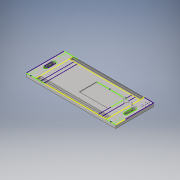
# Autodesk Inventor part: Button Fixture Base
Saved by Autodesk Inventor 2016 (Build 200138000, 138)
## iProperties
Created: 2016-07-07
Part Number: Button Fixture Base
Material: Generic
Document SubType Name: Modeling
Designer: Sam Clay
Density: 1 g/cm^3
Appearance: Default
Author: Sam Clay
Autodesk Inventor part; units mm, degrees
ref_plane "YZ Plane" through (0, 0, 0) normal (1, 0, 0) x (0, 1, 0)
ref_plane "XZ Plane" through (0, 0, 0) normal (0, 1, 0) x (-1, 0, 0)
ref_plane "XY Plane" through (0, 0, 0) normal (0, 0, 1) x (1, 0, 0)
sketch "Sketch1" plane through (0, 0, 0) normal (0, 1, 0) x (-1, 0, 0)
  line L0 (0, 0) -> (381, 0)
  line L1 (381, 0) -> (381, 203.2)
  line L2 (381, 203.2) -> (0, 203.2)
  line L3 (0, 203.2) -> (0, 0)
  line L4 (381, 0) -> (431.8, 0)
  line L5 (431.8, 0) -> (431.8, 203.2)
  line L6 (431.8, 203.2) -> (381, 203.2)
  line L7 (381, 203.2) -> (381, 0)
  line L8 (0, 0) -> (-50.8, 0)
  line L9 (-50.8, 0) -> (-50.8, 203.2)
  line L10 (-50.8, 203.2) -> (0, 203.2)
  line L11 (0, 203.2) -> (0, 0)
  dimension "d0" = 381
  dimension "d1" = 203.2
  dimension "d2" = 50.8
  dimension "d3" = 50.8
  constraints: 24 end point, 6 parallel, 3 horizontal, 3 perpendicular, 2 point on line
  measures "d0" distance of L2.end L1.end
  measures "d1" distance of L1.end L0.end
  measures "d2" distance of L6.end L5.end
  measures "d3" distance of L9.end L10.end
extrude "Extrusion1" add sketch "Sketch1" along normal blind 19.05 contours L3 L2 L1 L0
extrude "Extrusion2" add sketch "Sketch1" along normal blind 17.78 contours L8 L9 L10 L3 | L1 L6 L5 L4
sketch "Sketch2" plane through (0, 19.05, 0) normal (0, 1, 0) x (1, 0, 0)
  line L0 (-381, 0) -> (-381, -203.2) projected
  line L1 (0, 0) -> (-381, 0)
  line L2 (-381, 0) -> (-381, -3.175)
  line L3 (-381, -3.175) -> (0, -3.175)
  line L4 (0, -3.175) -> (0, 0)
  line L5 (0, -3.175) -> (-381, -3.175)
  line L6 (-381, -3.175) -> (-381, -22.987)
  line L7 (-381, -22.987) -> (0, -22.987)
  line L8 (0, -22.987) -> (0, -3.175)
  line L9 (0, -22.987) -> (-381, -22.987)
  line L10 (-381, -22.987) -> (-381, -54.737)
  line L11 (-381, -54.737) -> (0, -54.737)
  line L12 (0, -54.737) -> (0, -22.987)
  line L13 (0, -54.737) -> (-381, -54.737)
  line L14 (-381, -54.737) -> (-381, -148.717)
  line L15 (-381, -148.717) -> (0, -148.717)
  line L16 (0, -148.717) -> (0, -54.737)
  line L17 (0, -148.717) -> (-381, -148.717)
  line L18 (-381, -148.717) -> (-381, -180.467)
  line L19 (-381, -180.467) -> (0, -180.467)
  line L20 (0, -180.467) -> (0, -148.717)
  line L21 (0, -180.467) -> (-381, -180.467)
  line L22 (-381, -180.467) -> (-381, -200.279)
  line L23 (-381, -200.279) -> (0, -200.279)
  line L24 (0, -200.279) -> (0, -180.467)
  line L25 (0, -200.279) -> (-381, -200.279)
  line L26 (-381, -200.279) -> (-381, -203.454)
  line L27 (-381, -203.454) -> (0, -203.454)
  line L28 (0, -203.454) -> (0, -200.279)
  line L29 (0, -203.2) -> (0, 0) projected
  line L30 (0, 0) -> (-44.45, 0)
  line L31 (-44.45, 0) -> (-44.45, -148.717)
  line L32 (-44.45, -148.717) -> (0, -148.717)
  line L33 (0, -148.717) -> (0, 0)
  circle A0 centre (-48.1046, -57.912) radius 8.89
  line L34 (-44.45, -54.737) -> (-199.39, -54.737)
  line L35 (-199.39, -54.737) -> (-199.39, -148.717)
  line L36 (-199.39, -148.717) -> (-44.45, -148.717)
  line L37 (-44.45, -148.717) -> (-44.45, -54.737)
  dimension "d8" = 3.175
  dimension "d9" = 19.812
  dimension "d10" = 31.75
  dimension "d11" = 93.98
  dimension "d12" = 31.75
  dimension "d13" = 19.812
  dimension "d14" = 3.175
  dimension "d15" = 44.45
  dimension "d16" = 17.78
  dimension "d21" = 3.175
  dimension "d49" = 154.94
  constraints: 72 end point, 18 parallel, 11 point on line, 9 horizontal, 9 perpendicular, 1 centre point
  measures "d8" distance of L2.end L1.end
  measures "d9" distance of L6.end L5.end
  measures "d10" distance of L10.end L9.end
  measures "d11" distance of L14.end L13.end
  measures "d12" distance of L18.end L17.end
  measures "d13" distance of L22.end L21.end
  measures "d14" distance of L26.end L25.end
  measures "d15" distance of L32.end L31.end
  measures "d16" diameter of A0
  measures "d21" distance from line of L13 A0.centre
  measures "d49" distance of L36.end L35.end
extrude "Extrusion3" cut sketch "Sketch2" against normal blind 11.43 contours L3 L31 L7 L0 | L3 L8 L7 L31 | L19 L24 L23 L0
extrude "Extrusion4" cut sketch "Sketch2" against normal blind 1.651 contours L11 A0 L31 L15 L35 | A0 L11 L31 | L31 L11 A0 | L11 L31 A0 | L11 A0 L31
sketch "Sketch3" plane through (0, 19.05, 0) normal (0, 1, 0) x (1, 0, 0)
  line L0 (50.8, -152.4) -> (50.8, 0)
  line L1 (50.8, 0) -> (0, 0)
  line L2 (-431.8, 0) -> (-431.8, -152.4)
  line L3 (-355.6, 0) -> (-431.8, 0)
  line L4 (-431.8, -203.2) -> (-330.2, -203.2)
  line L5 (-406.4, -79.375) -> (-406.4, -123.825) construction
  line L6 (-415.925, -79.375) -> (-415.925, -123.825)
  line L7 (-396.875, -123.825) -> (-396.875, -79.375)
  arc A0 (-396.875, -79.375) -> (-415.925, -79.375) centre (-406.4, -79.375) ccw
  arc A1 (-415.925, -123.825) -> (-396.875, -123.825) centre (-406.4, -123.825) ccw
  line L8 (25.4, -79.375) -> (25.4, -123.825) construction
  line L9 (15.875, -79.375) -> (15.875, -123.825)
  line L10 (34.925, -123.825) -> (34.925, -79.375)
  arc A2 (34.925, -79.375) -> (15.875, -79.375) centre (25.4, -79.375) ccw
  arc A3 (15.875, -123.825) -> (34.925, -123.825) centre (25.4, -123.825) ccw
  line L11 (-177.8, -54.737) -> (-37.282, -54.737)
  line L12 (-44.45, -46.3991) -> (-44.45, -117.636)
  line L13 (-431.8, -203.2) -> (-381, -203.2)
  line L14 (0, -203.2) -> (50.8, -203.2)
  line L15 (50.8, 0) -> (0, 0)
  line L16 (50.8, -152.4) -> (50.8, 0)
  line L17 (-431.8, 0) -> (-431.8, -203.2)
  line L18 (-199.39, -54.737) -> (-56.4083, -54.737)
  line L19 (-44.45, -66.0161) -> (-44.45, -136.017)
  line L20 (-199.39, -54.737) -> (-56.4083, -54.737) projected
  line L21 (-44.45, -66.0161) -> (-44.45, -148.717) projected
  line L22 (-381, 0) -> (-431.8, 0) projected
  line L23 (-431.8, 0) -> (-431.8, -203.2) projected
  line L24 (-431.8, -203.2) -> (-381, -203.2) projected
  line L25 (-381, -200.279) -> (-381, -203.2) projected
  line L26 (-381, -180.467) -> (-381, -200.279) projected
  line L27 (-381, -22.987) -> (-381, -180.467) projected
  line L28 (-381, -3.175) -> (-381, -22.987) projected
  line L29 (-381, 0) -> (-381, -3.175) projected
  line L30 (0, -203.2) -> (0, -200.279) projected
  line L31 (0, -203.2) -> (50.8, -203.2) projected
  line L32 (50.8, -203.2) -> (50.8, 0) projected
  line L33 (50.8, 0) -> (0, 0) projected
  line L34 (0, -3.175) -> (0, 0) projected
  line L35 (0, -22.987) -> (0, -3.175) projected
  line L36 (0, -180.467) -> (0, -22.987) projected
  line L37 (0, -200.279) -> (0, -180.467) projected
  point P0 (-44.45, -54.737)
  point P1 (38.1, -19.05)
  point P2 (38.1, -38.1)
  point P3 (38.1, -180.467)
  point P4 (38.1, -161.417)
  point P5 (-419.1, -19.05)
  point P6 (-419.1, -38.1)
  point P7 (-419.1, -184.15)
  point P8 (-419.1, -165.1)
  point P9 (-406.4, -101.6)
  point P10 (25.4, -101.6)
  point P11 (-127.8992, -54.737)
  point P12 (-406.4, -203.2)
  point P13 (25.4, -203.2)
  dimension "d22" = 12.7
  dimension "d23" = 19.05
  dimension "d25" = 12.7
  dimension "d26" = 19.05
  dimension "d27" = 19.05
  dimension "d28" = 12.7
  dimension "d29" = 12.7
  dimension "d30" = 12.7
  dimension "d31" = 19.05
  dimension "d33" = 19.05
  dimension "d34" = 19.05
  dimension "d35" = 19.05
  dimension "d36" = 12.7
  dimension "d37" = 12.7
  dimension "d38" = 12.7
  dimension "d39" = 44.45
  dimension "d40" = 19.05
  dimension "d43" = 44.45
  dimension "d44" = 19.05
  dimension "d53" = 25.4
  constraints: 44 end point, 8 point on circle, 8 tangent, 7 midpoint, 6 collinear, 4 centre point, 4 point on line, 2 parallel, 2 vertical, 5 other
  measures "d22" distance from line of L0 point (38.1, -19.05)
  measures "d23" distance from line of L1 point (38.1, -19.05)
  measures "d25" distance from line of L0 point (38.1, -180.467)
  measures "d26" distance of point (38.1, -38.1) point (38.1, -19.05)
  measures "d27" distance of point (38.1, -161.417) point (38.1, -180.467)
  measures "d28" distance from line of L0 point (38.1, -161.417)
  measures "d29" distance from line of L0 point (38.1, -38.1)
  measures "d30" distance from line of L2 point (-419.1, -19.05)
  measures "d31" distance from line of L3 point (-419.1, -19.05)
  measures "d33" distance of point (-419.1, -19.05) point (-419.1, -38.1)
  measures "d34" distance of point (-419.1, -184.15) point (-419.1, -165.1)
  measures "d35" distance from line of L4 point (-419.1, -184.15)
  measures "d36" distance from line of L2 point (-419.1, -38.1)
  measures "d37" distance from line of L2 point (-419.1, -165.1)
  measures "d38" distance from line of L2 point (-419.1, -184.15)
  measures "d39" distance of L5.start L5.end
  measures "d40" diameter of A1
  measures "d43" distance of L8.start L8.end
  measures "d44" diameter of A3
  measures "d53" distance from line of point (-406.4, -101.6) L2
extrude "Extrusion5" cut sketch "Sketch3" against normal through all contours A0 L7 A1 L6 | A2 L10 A3 L9
sketch "Sketch4" plane through (0, 19.05, 0) normal (0, 1, 0) x (1, 0, 0)
  line L0 (0, -22.987) -> (-381, -22.987) projected
  line L1 (-355.6, -22.987) -> (-355.6, -203.2)
  line L2 (-25.4, -22.987) -> (-25.4, -203.2)
  line L3 (-381, -22.987) -> (-381, -3.175) projected
  line L4 (0, -203.2) -> (0, -22.987) projected
  line L5 (-336.55, -22.987) -> (-336.55, -203.2)
  line L6 (-381, -203.2) -> (0, -203.2) projected
  line L7 (-44.45, -22.987) -> (-44.45, -203.2)
  point P0 (0, 0)
  dimension "d50" = 25.4
  dimension "d51" = 25.4
  dimension "d52" = 19.05
  dimension "d55" = 19.05
  constraints: 8 end point, 8 point on line, 2 vertical, 1 parallel
  measures "d50" distance between parallel lines of L1 L3
  measures "d51" distance between parallel lines of L2 L4
  measures "d52" distance between parallel lines of L5 L1
  measures "d55" distance between parallel lines of L7 L2
equation "\"d13\" = d9"
equation "\"d25\" = d22"
equation "\"d26\" = d23"
equation "\"d27\" = d26"
equation "\"d28\" = d22"
equation "\"d29\" = d22"
equation "\"d30\" = d22"
equation "\"d31\" = d23"
equation "\"d33\" = d31"
equation "\"d34\" = d31"
equation "\"d35\" = d31"
equation "\"d36\" = d22"
equation "\"d37\" = d22"
equation "\"d38\" = d22"
equation "\"d39\" = d43"
equation "\"d40\" = d44"
body "Solid1"
